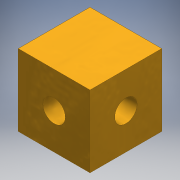
# Autodesk Inventor part: 垂直ブロック 真鍮 8
Saved by Autodesk Inventor 2020.2 (Build 242310000, 310)
## iProperties
Created: 2019-03-21
Part Number: 垂直ブロック 真鍮 8
Material: 真鍮、ソフト イエロー
Document SubType Name: Modeling
Designer: mozar
Density: 8.47 g/cm^3
Appearance: 溶接 - 真鍮
Author: mozar
Autodesk Inventor part; units mm, degrees
ref_plane "YZ Plane" through (0, 0, 0) normal (1, 0, 0) x (0, 1, 0)
ref_plane "XZ Plane" through (0, 0, 0) normal (0, 1, 0) x (-1, 0, 0)
ref_plane "XY Plane" through (0, 0, 0) normal (0, 0, 1) x (1, 0, 0)
sketch "スケッチ1" plane through (0, 0, 0) normal (0, 0, 1) x (1, 0, 0)
  line L0 (0, 0) -> (8, 0)
  line L1 (8, 0) -> (8, -8)
  line L2 (8, -8) -> (0, -8)
  line L3 (0, -8) -> (0, 0)
  line L4 (0, -4) -> (8, -4)
  line L5 (4, 0) -> (4, -8)
  dimension "d0" = 8
  dimension "d1" = 8
  constraints: 12 end point, 4 midpoint, 2 parallel, 1 horizontal, 1 perpendicular
  measures "d0" distance of L1.end L2.end
  measures "d1" distance of L0.end L1.end
extrude "押し出し1" add sketch "スケッチ1" along normal blind 8
sketch "スケッチ2" plane through (8, -8, 0) normal (1, 0, 0) x (0, 0, -1)
  line L0 (-8, 8) -> (0, 8) projected
  line L1 (0, 8) -> (0, 0) projected
  line L2 (0, 0) -> (-8, 0) projected
  line L3 (-8, 0) -> (-8, 8) projected
  line L4 (-8, 8) -> (0, 0)
  line L5 (0, 8) -> (0, 0) projected
  line L6 (-8, 0) -> (0, 8)
  point P0 (-4, 4)
  constraints: 4 end point, 1 midpoint
hole "穴1" at (8, -4, 4) direction (-1, 0, 0) diameter 2.5 end through all
sketch "スケッチ3" plane through (0, 0, 0) normal (0, 1, 0) x (1, 0, 0)
  line L0 (8, 0) -> (8, -8) projected
  line L1 (8, -8) -> (0, -8) projected
  line L2 (0, -8) -> (0, 0) projected
  line L3 (0, 0) -> (8, 0) projected
  line L4 (0, -8) -> (8, 0)
  line L5 (8, 0) -> (8, -8) projected
  line L6 (0, 0) -> (8, 0) projected
  line L7 (8, -8) -> (0, 0)
  point P0 (4, -4)
  constraints: 4 end point, 1 midpoint, 1 perpendicular
hole "穴2" at (4, 0, 4) direction (0, -1, 0) diameter 2.5 end through all
equation "\"d0\" = d1"
